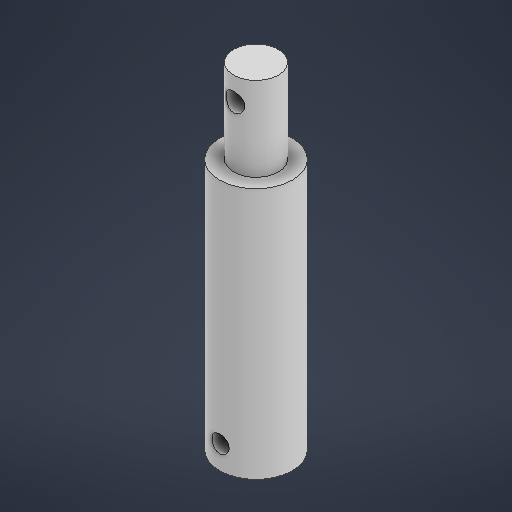
# Autodesk Inventor part: Lego-Frame-Holder-Extra-Extra
Saved by Autodesk Inventor 2025 (Build 290162010, 162A)
## iProperties
Created: 2024-06-29
Part Number: Lego-Frame-Holder-Extra-Extra
Material: Generic
Document SubType Name: Modeling
Designer: Windows 11
Density: 1 g/cm^3
Appearance: Default
Author: Windows 11
Autodesk Inventor part; units mm, degrees
ref_plane "YZ Plane" through (0, 0, 0) normal (1, 0, 0) x (0, 1, 0)
ref_plane "XZ Plane" through (0, 0, 0) normal (0, 1, 0) x (-1, 0, 0)
ref_plane "XY Plane" through (0, 0, 0) normal (0, 0, 1) x (1, 0, 0)
sketch "Sketch1" plane through (0, 0, 0) normal (0, 1, 0) x (-1, 0, 0)
  circle A0 centre (0, 0) radius 3.9
  dimension "d0" = 7.8
  constraints: 1 centre point, 1 coincident
  measures "d0" diameter of A0
extrude "Extrusion1" add sketch "Sketch1" along normal blind 27
sketch "Sketch2" plane through (0, 27, 0) normal (0, 1, 0) x (1, 0, 0)
  circle A0 centre (0, 0) radius 2.4
  dimension "d3" = 4.8
  constraints: 1 centre point, 1 coincident
  measures "d3" diameter of A0
extrude "Extrusion2" add sketch "Sketch2" along normal blind 9
sketch "Sketch3" plane through (0, 0, 0) normal (0, -1, 0) x (1, 0, 0)
  circle A0 centre (0, 0) radius 2.4
  dimension "d6" = 4.8
  constraints: 1 centre point, 1 coincident
  measures "d6" diameter of A0
extrude "Extrusion3" cut sketch "Sketch3" against normal blind 5
sketch "Sketch4" plane through (0, 0, 0) normal (0, 1, 0) x (-1, 0, 0)
  line L0 (0, 0) -> (0, 3.9)
  circle A0 centre (0, 0) radius 3.9 projected
  constraints: 2 end point, 1 coincident, 1 vertical, 1 vertical alignment, 1 other
ref_plane "Work Plane1" through (0, 0, 3.9) normal (0, 0, 1) x (1, 0, 0)
sketch "Sketch5" plane through (0, 0, 3.9) normal (0, 0, 1) x (1, 0, 0)
  line L0 (0, 0) -> (0, 2.5)
  dimension "d9" = 2.5
  constraints: 2 end point, 1 coincident, 1 vertical
  measures "d9" distance of L0.start L0.end
hole "Hole1" at (0, 2.5, 3.9) direction (0, 0, -1) diameter 1.854 end through all clearance for "Flat Head Machine Screw (82)" size "#0" standard "Ansi Unified Screw Threads"
sketch "Sketch6" plane through (0, 0, 3.9) normal (0, 0, 1) x (1, 0, 0)
  line L0 (0, 0) -> (0, 27)
  line L1 (3.9, 27) -> (-3.9, 27) projected
  line L2 (0, 27) -> (0, 33.5)
  dimension "d17" = 6.5
  constraints: 4 end point, 1 coincident, 1 midpoint, 1 point on line
  measures "d17" distance of L0.end L2.end
hole "Hole2" at (0, 33.5, 3.9) direction (0, 0, -1) diameter 2 end through all clearance for "Flat Head Machine Screw (82)" size "#0" standard "Ansi Unified Screw Threads"
body "Solid1"
